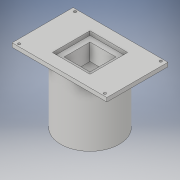
# Autodesk Inventor part: spad_sensor_tube_long_istvan
Saved by Autodesk Inventor 2018 (Build 220112000, 112)
## iProperties
Created: 2017-08-18
Part Number: spad_sensor_tube_long_istvan
Material: Generic
Document SubType Name: Modeling
Designer: s1158328
Density: 1 g/cm^3
Appearance: Default
Author: s1158328
Autodesk Inventor part; units mm, degrees
ref_plane "XZ Plane" through (0, 0, 0) normal (0, 1, 0) x (-1, 0, 0)
ref_plane "XY Plane" through (0, 0, 0) normal (0, 0, 1) x (1, 0, 0)
sketch "Sketch1" plane through (0, 0, 0) normal (0, 1, 0) x (-1, 0, 0)
  line L0 (-10, -10) -> (10, -10)
  line L1 (10, -10) -> (10, 10)
  line L2 (10, 10) -> (-10, 10)
  line L3 (-10, 10) -> (-10, -10)
  line L4 (-10, -10) -> (10, 10) construction
  line L5 (10, -10) -> (-10, 10) construction
  circle A0 centre (0, 0) radius 19.5
  dimension "d0" = 20
  dimension "d1" = 39
  constraints: 12 end point, 2 midpoint, 2 parallel, 1 centre point, 1 coincident, 1 horizontal, 1 perpendicular
  measures "d0" distance of L0.end L1.end
  measures "d1" diameter of A0
extrude "Extrusion1" add sketch "Sketch1" along normal blind 10
sketch "Sketch8" plane through (0, 10, 0) normal (0, 1, 0) x (1, 0, 0)
  line L0 (10, -10) -> (-10, -10) projected
  line L1 (-10, 10) -> (10, 10) projected
  line L2 (-20, 16) -> (26, 16)
  line L3 (26, 16) -> (26, -16)
  line L4 (26, -16) -> (-20, -16)
  line L5 (-20, -16) -> (-20, 16)
  line L6 (-10, -10) -> (-10, 10) projected
  line L7 (14.5, -14.2875) -> (-14.5, -14.2875)
  line L8 (-14.5, -14.2875) -> (-14.5, 14.2875)
  line L9 (-14.5, 14.2875) -> (14.5, 14.2875)
  line L10 (14.5, 14.2875) -> (14.5, -14.2875)
  line L11 (14.5, -14.2875) -> (-14.5, 14.2875) construction
  line L12 (-14.5, -14.2875) -> (14.5, 14.2875) construction
  point P0 (0, 0)
  dimension "d23" = 20
  dimension "d24" = 10
  dimension "d25" = 6
  dimension "d26" = 6
  dimension "d27" = 46
  dimension "d30" = 29
  constraints: 20 end point, 4 parallel, 2 midpoint, 2 perpendicular, 1 horizontal
  measures "d23" distance between parallel lines of L0 L1
  measures "d24" distance between parallel lines of L5 L6
  measures "d25" distance between parallel lines of L1 L2
  measures "d26" distance between parallel lines of L4 L0
  measures "d27" distance between parallel lines of L3 L5
  measures "d30" distance of L8.end L9.end
extrude "Extrusion5" add sketch "Sketch8" along normal blind 6 contours L2 L3 L4 L5 | L7 L8 L9 L10
sketch "Sketch9" plane through (0, 16, 0) normal (0, 1, 0) x (1, 0, 0)
  line L0 (14.5, 14.5) -> (-14.5, 14.5)
  line L1 (-14.5, 14.5) -> (-14.5, -14.5)
  line L2 (-14.5, -14.5) -> (14.5, -14.5)
  line L3 (14.5, -14.5) -> (14.5, 14.5)
  line L4 (14.5, 14.5) -> (-14.5, -14.5) construction
  line L5 (-14.5, 14.5) -> (14.5, -14.5) construction
  point P0 (0, 0)
  dimension "d31" = 29
  dimension "d32" = 29
  constraints: 12 end point, 2 midpoint, 2 parallel, 1 horizontal, 1 perpendicular
  measures "d31" distance of L0.end L1.end
  measures "d32" distance of L0.start L0.end
extrude "Extrusion6" cut sketch "Sketch9" against normal blind 3
sketch "Sketch10" plane through (0, 13, 0) normal (0, 1, 0) x (1, 0, 0)
  line L0 (10, -10) -> (-10, -10) projected
  line L1 (10, 10) -> (-10, 10)
  line L2 (-10, 10) -> (-10, -10)
  line L3 (-10, -10) -> (10, -10)
  line L4 (10, -10) -> (10, 10)
  line L5 (10, 10) -> (-10, -10) construction
  line L6 (-10, 10) -> (10, -10) construction
  point P0 (0, 0)
  dimension "d35" = 20
  dimension "d36" = 20
  constraints: 12 end point, 2 midpoint, 2 parallel, 1 horizontal, 1 perpendicular
  measures "d35" distance of L1.end L0.end
  measures "d36" distance of L1.start L1.end
extrude "Extrusion7" cut sketch "Sketch10" against normal blind 5
ref_plane "Work Plane2" through (-20, 0, 0) normal (1, 0, 0) x (0, 1, 0)
sketch "Sketch12" plane through (0, 16, 0) normal (0, 1, 0) x (1, 0, 0)
  line L0 (36.5, -23.5) -> (36.5, 23.5)
  line L1 (36.5, 23.5) -> (-36.5, 23.5)
  line L2 (-36.5, 23.5) -> (-36.5, -23.5)
  line L3 (-36.5, -23.5) -> (36.5, -23.5)
  line L4 (-20, -16) -> (26, -16) projected
  line L5 (26, 16) -> (-20, 16) projected
  line L6 (14.5, -14.5) -> (-14.5, -14.5) projected
  line L7 (-14.5, -14.5) -> (-14.5, 14.5) projected
  line L8 (14.5, 14.5) -> (14.5, -14.5) projected
  line L9 (-14.5, 14.5) -> (14.5, 14.5) projected
  line L10 (-14.5, 14.5) -> (14.5, 14.5)
  line L11 (14.5, 14.5) -> (14.5, -14.5)
  line L12 (14.5, -14.5) -> (-14.5, -14.5)
  line L13 (-14.5, -14.5) -> (-14.5, 14.5)
  line L14 (-14.5, 14.5) -> (14.5, -14.5) construction
  line L15 (14.5, 14.5) -> (-14.5, -14.5) construction
  point P0 (0, 0)
  dimension "d48" = 7.5
  dimension "d49" = 7.5
  dimension "d50" = 9
  dimension "d51" = 22
  dimension "d52" = 22
  dimension "d53" = 73
  dimension "d54" = 9
  dimension "d55" = 29
  constraints: 20 end point, 4 parallel, 2 midpoint, 2 perpendicular, 1 horizontal, 1 vertical
  measures "d48" distance between parallel lines of L3 L4
  measures "d49" distance between parallel lines of L1 L5
  measures "d50" distance between parallel lines of L3 L6
  measures "d51" distance between parallel lines of L2 L7
  measures "d52" distance between parallel lines of L0 L8
  measures "d53" distance between parallel lines of L2 L0
  measures "d54" distance between parallel lines of L9 L1
  measures "d55" distance between parallel lines of L9 L6
extrude "Extrusion9" add sketch "Sketch12" against normal blind 3
sketch "Sketch13" plane through (0, 16, 0) normal (0, 1, 0) x (1, 0, 0)
  circle A0 centre (33, -21.5) radius 1
  line L0 (36.5, -23.5) -> (36.5, 23.5) projected
  line L1 (-36.5, -23.5) -> (36.5, -23.5) projected
  line L2 (36.5, 23.5) -> (-36.5, 23.5) projected
  point P0 (0, 0)
  dimension "d58" = 2
  dimension "d59" = 3.5
  dimension "d60" = 2
  dimension "d61" = 47
  constraints: 1 centre point
  measures "d58" diameter of A0
  measures "d59" distance from line of L0 A0.centre
  measures "d60" distance from line of L1 A0.centre
  measures "d61" distance between parallel lines of L2 L1
extrude "Extrusion10" cut sketch "Sketch13" against normal blind 3
sketch "Sketch14" plane through (0, 16, 0) normal (0, 1, 0) x (1, 0, 0)
  circle A0 centre (33, 21.5) radius 1
  line L0 (36.5, -23.5) -> (36.5, 23.5) projected
  line L1 (36.5, 23.5) -> (-36.5, 23.5) projected
  point P0 (0, 0)
  dimension "d64" = 2
  dimension "d65" = 3.5
  dimension "d66" = 2
  constraints: 1 centre point
  measures "d64" diameter of A0
  measures "d65" distance from line of L0 A0.centre
  measures "d66" distance from line of L1 A0.centre
extrude "Extrusion11" cut sketch "Sketch14" against normal blind 3
sketch "Sketch15" plane through (0, 16, 0) normal (0, 1, 0) x (1, 0, 0)
  circle A0 centre (-33, -21.5) radius 1
  line L0 (-36.5, 23.5) -> (-36.5, -23.5) projected
  line L1 (-36.5, -23.5) -> (36.5, -23.5) projected
  point P0 (0, 0)
  dimension "d69" = 2
  dimension "d70" = 3.5
  dimension "d71" = 2
  constraints: 1 centre point
  measures "d69" diameter of A0
  measures "d70" distance from line of L0 A0.centre
  measures "d71" distance from line of L1 A0.centre
extrude "Extrusion12" cut sketch "Sketch15" against normal blind 3
sketch "Sketch16" plane through (0, 16, 0) normal (0, 1, 0) x (1, 0, 0)
  circle A0 centre (-33, 21.5) radius 1
  line L0 (-36.5, 23.5) -> (-36.5, -23.5) projected
  line L1 (36.5, 23.5) -> (-36.5, 23.5) projected
  point P0 (0, 0)
  dimension "d74" = 2
  dimension "d75" = 3.5
  dimension "d76" = 2
  constraints: 1 centre point
  measures "d74" diameter of A0
  measures "d75" distance from line of L0 A0.centre
  measures "d76" distance from line of L1 A0.centre
extrude "Extrusion13" cut sketch "Sketch16" against normal blind 3
sketch "Sketch17" plane through (0, 10, 0) normal (0, -1, 0) x (1, 0, 0)
  circle A0 centre (0, 0) radius 22.5
  circle A1 centre (0, 0) radius 19.5
  dimension "d79" = 45
  dimension "d80" = 39
  constraints: 2 centre point, 2 coincident
  measures "d79" diameter of A0
  measures "d80" diameter of A1
extrude "Extrusion14" add sketch "Sketch17" along normal blind 44 and the other way blind 3
body "Solid1"
